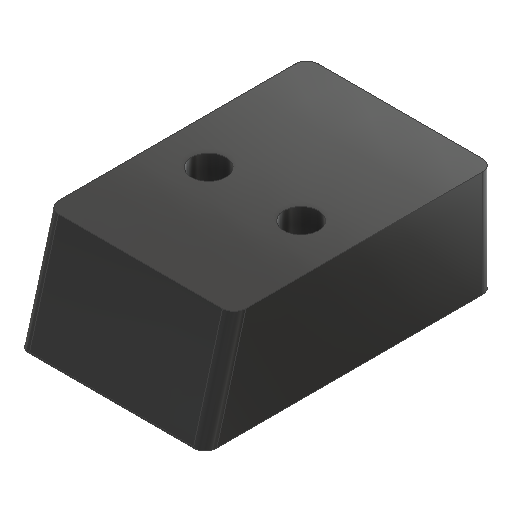
# Autodesk Inventor part: 3DP_ABS_X_Axis_IGUS_Cable_Chain_Mount
Saved by Autodesk Inventor 2026.1 (Build 301233000, 233)
## iProperties
Created: 2016-06-18
Part Number: 3DP_ABS_X_Axis_IGUS_Cable_Chain_Mount
Material: Ogólny
Document SubType Name: Modeling
Designer: Andrzej
Density: 1 g/cm^3
Appearance: Ciemnoszara
Mass: 3.57754 g
Surface Area: 16.8766 cm^2
Volume: 3.57754 cm^3
Author: Andrzej
Autodesk Inventor part; units mm, degrees
ref_plane "YZ Plane" through (0, 0, 0) normal (1, 0, 0) x (0, 1, 0)
ref_plane "XZ Plane" through (0, 0, 0) normal (0, 1, 0) x (-1, 0, 0)
ref_plane "XY Plane" through (0, 0, 0) normal (0, 0, 1) x (1, 0, 0)
sketch "Szkic1" plane through (0, 0, 0) normal (0, 0, 1) x (1, 0, 0)
  line L0 (-10.8514, 21.0596) -> (5.3486, 21.0596)
  line L1 (5.3486, 21.0596) -> (5.3486, -3.9404)
  line L2 (5.3486, -3.9404) -> (-10.8514, -3.9404)
  line L3 (-10.8514, -3.9404) -> (-10.8514, 21.0596)
  point P0 (0, 0)
  dimension "d0" = 16.2
  dimension "d1" = 25
  constraints: 8 end point, 2 parallel, 1 horizontal, 1 perpendicular
  measures "d0" distance of L1.end L2.end
  measures "d1" distance of L0.end L1.end
extrude "Wyciągnięcie proste1" add sketch "Szkic1" along normal blind 9.2
sketch "Szkic2" plane through (0, 0, 9.2) normal (0, 0, 1) x (1, 0, 0)
  line L0 (5.3486, 21.0596) -> (-10.8514, 21.0596) projected
  line L1 (-10.8514, 21.0596) -> (-10.8514, -3.9404) projected
  line L2 (-10.8514, -3.9404) -> (5.3486, -3.9404) projected
  line L3 (5.3486, -3.9404) -> (5.3486, 21.0596) projected
  point P0 (0, 0)
  point P1 (-6.8514, 8.5596)
  point P2 (1.1486, 8.5596)
  dimension "d4" = 12.5
  dimension "d5" = 12.5
  dimension "d6" = 4
  dimension "d7" = 4.2
  measures "d4" distance from line of L0 point (-6.851, 8.56)
  measures "d5" distance from line of L0 point (1.149, 8.56)
  measures "d6" distance from line of L1 point (-6.851, 8.56)
  measures "d7" distance from line of L3 point (1.149, 8.56)
hole "Otwór1" at (-6.8514, 8.5596, 9.2) at (1.1486, 8.5596, 9.2) direction (0, 0, -1) diameter 3 end through all
chamfer "Faza3" distance 2.5 distance2 9.1 1 edges at (-2.7514, -3.9404, 9.2) measured on face at (-1.6837, 17.3356, 9.2)
fillet "Zaokrąglenie1" radius 1 4 edges at (-10.8514, 21.0596, 4.6) (5.3486, -2.6904, 4.65) (-10.8514, -2.6904, 4.65) (5.3486, 21.0596, 4.6)
equation "\"d5\" = d4"
